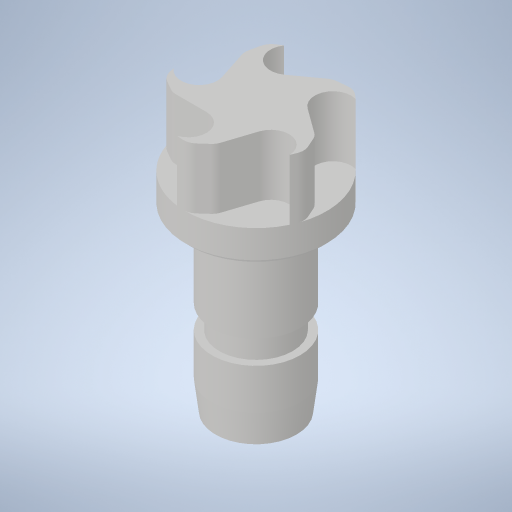
# Autodesk Inventor part: 2.5mm_uncorrected
Saved by Autodesk Inventor 2023.1 (Build 271208000, 208)
## iProperties
Created: 2020-02-22
Part Number: 2.5mm_uncorrected
Material: Generic
Document SubType Name: Modeling
Designer: kongooi
Density: 1 g/cm^3
Appearance: Default
Author: kongooi
Autodesk Inventor part; units mm, degrees
ref_plane "YZ Plane" through (0, 0, 0) normal (1, 0, 0) x (0, 1, 0)
sketch "Sketch2" plane through (0, 0, 0) normal (0, 1, 0) x (-1, 0, 0)
  line L0 (-0.2546, 1.0207) -> (-0.1225, 1.1396)
  line L1 (-0.2546, 1.0207) -> (-0.1225, 1.1396)
  line L2 (-0.3944, -0.9754) -> (-0.571, -0.9938)
  arc A0 (0.5758, -1.0527) -> (0.139, -0.6263) centre (0.3209, -0.8769) ccw
  line L3 (-0.2826, -0.9325) -> (0.139, -0.6263)
  arc A1 (-0.8233, -0.873) -> (-0.7386, -0.9457) centre (-0.0001, 0.0001) ccw
  line L4 (-0.2826, -0.9325) -> (0.139, -0.6263)
  arc A2 (-0.3944, -0.9754) -> (-0.2826, -0.9325) centre (-0.4184, -0.7455) ccw
  line L5 (0.8922, 0.5575) -> (1.046, 0.4685)
  arc A3 (0.1528, 1.1903) -> (0.2557, 0.5886) centre (0.2557, 0.8982) ccw
  line L6 (0.7766, 0.5885) -> (0.2557, 0.5886)
  arc A4 (0.8922, 0.5575) -> (0.7766, 0.5885) centre (0.7766, 0.3574) ccw
  line L7 (0.8057, -0.6769) -> (0.7687, -0.8501)
  arc A5 (1.1791, 0.2224) -> (0.6381, -0.0606) centre (0.9326, 0.035) ccw
  line L8 (0.7994, -0.5574) -> (0.6381, -0.0606)
  arc A6 (0.8057, -0.6769) -> (0.7994, -0.5574) centre (0.5796, -0.6287) ccw
  arc A7 (-1.0848, 0.5133) -> (-0.4808, 0.4252) centre (-0.7752, 0.5209) ccw
  line L9 (-0.3197, 0.9205) -> (-0.4808, 0.4252)
  arc A8 (-0.2546, 1.0207) -> (-0.3197, 0.9205) centre (-0.1, 0.849) ccw
  line L10 (-1.0496, 0.0736) -> (-1.1218, 0.2359)
  arc A9 (-0.8233, -0.873) -> (-0.5529, -0.3258) centre (-0.7349, -0.5763) ccw
  line L11 (-0.9743, -0.0195) -> (-0.5529, -0.3258)
  arc A10 (-1.0496, 0.0736) -> (-0.9743, -0.0195) centre (-0.8385, 0.1675) ccw
  arc A11 (1.1791, 0.2224) -> (1.1534, 0.3311) centre (-0.0001, 0.0001) ccw
  arc A12 (-1.0848, 0.5133) -> (-1.1278, 0.4102) centre (-0.0001, 0.0001) ccw
  arc A13 (0.5758, -1.0527) -> (0.6712, -0.9946) centre (-0.0001, 0.0001) ccw
  arc A14 (0.1528, 1.1903) -> (0.0414, 1.1993) centre (-0.0001, 0.0001) ccw
  arc A15 (0.0414, 1.1993) -> (-0.1225, 1.1396) centre (0.0334, 0.9665) ccw
  arc A16 (-1.1278, 0.4102) -> (-1.1218, 0.2359) centre (-0.9089, 0.3305) ccw
  arc A17 (1.1534, 0.3311) -> (1.046, 0.4685) centre (0.9294, 0.2668) ccw
  arc A18 (-0.7386, -0.9457) -> (-0.571, -0.9938) centre (-0.5953, -0.7621) ccw
  arc A19 (0.6712, -0.9946) -> (0.7687, -0.8501) centre (0.5409, -0.8015) ccw
  circle A20 centre (-0.0001, 0.0001) radius 1.2
  point P0 (-1.0498, 0.074)
  point P1 (0.7767, 0.5884)
  point P2 (0.2555, 0.5884)
  dimension "d305" = 2.4
  constraints: 49 point on circle, 26 tangent, 24 end point, 20 centre point, 12 equal radius, 2 coincident, 2 collinear, 3 other
sketch "Sketch3" plane through (0, 0, 0) normal (0, 1, 0) x (-1, 0, 0)
  line L0 (5.0133, 39.043) -> (38.6813, 7.297)
  line L1 (38.6813, 7.297) -> (18.893, -34.5332)
  line L2 (18.893, -34.5332) -> (-27.0048, -28.6397)
  line L3 (-27.0048, -28.6397) -> (-35.5829, 16.8329)
  line L4 (-35.5829, 16.8329) -> (5.0133, 39.043)
  circle A0 centre (0, 0) radius 39.3635
  circle A1 centre (0, 0) radius 20.4353
  circle A2 centre (0, 0) radius 31.8458
  circle A3 centre (10.4717, -28.7325) radius 10.093
  circle A4 centre (41.1153, -0.5956) radius 4.0726
  circle A5 centre (8.144, 29.3283) radius 10.0252
  circle A6 centre (-25.3778, 16.9956) radius 10.0583
  circle A7 centre (-24.1576, -18.872) radius 10.1582
  line L5 (-25.3778, 16.9956) -> (8.3216, 29.3877)
  line L6 (8.3216, 29.3877) -> (30.5209, 1.1669)
  line L7 (30.5209, 1.1669) -> (10.5413, -28.6665)
  line L8 (10.5413, -28.6665) -> (-24.006, -18.8838)
  line L9 (-24.006, -18.8838) -> (-25.3778, 16.9956)
  line L10 (-31.306, -23.8626) -> (-32.3687, 22.3998)
  line L11 (-32.3687, 22.3998) -> (11.301, 37.7064)
  line L12 (11.301, 37.7064) -> (39.3531, 0.904)
  line L13 (39.3531, 0.904) -> (13.0206, -37.1477)
  line L14 (13.0206, -37.1477) -> (-31.306, -23.8626)
  point P0 (-9.1427, -30.5051)
  constraints: 30 end point, 6 centre point, 6 coincident, 4 tangent, 1 midpoint, 43 other
extrude "Extrusion4" add sketch "Sketch2" against normal blind 1.032 contours L0 A15 A14 A3 L6 A4 L5 A17 A11 A5 L8 A6 L7 A19 A13 A0 L3 A2 L2 A18 A1 A9 L11 A10 L10 A16 A12 A7 L9 A8
sketch "Sketch6" plane through (0, -1.032, 0) normal (0, -1, 0) x (1, 0, 0)
  circle A0 centre (0, 0) radius 1.2
  dimension "d304" = 2.4
  constraints: 1 centre point, 1 coincident
  measures "d304" diameter of A0
extrude "Extrusion5" add sketch "Sketch6" along normal blind 0.55
ref_plane "Plan de construction1" through (0, -1.582, 0) normal (0, -1, 0) x (1, 0, 0)
sketch "Sketch7" plane through (0, -1.582, 0) normal (0, -1, 0) x (1, 0, 0)
  circle A0 centre (0, 0) radius 0.75
  circle A1 centre (0, 0) radius 0.3
  circle A2 centre (0, 0) radius 0.625
  dimension "d303" = 1.5
  dimension "d306" = 0.6
  dimension "d307" = 1.25
  constraints: 3 centre point, 2 coincident
  measures "d303" diameter of A0
  measures "d306" diameter of A1
  measures "d307" diameter of A2
extrude "Extrusion6" add sketch "Sketch7" along normal blind 3 contours A0 | A2
ref_plane "Plan de construction2" through (0, -2.982, 0) normal (0, -1, 0) x (1, 0, 0)
extrude "Extrusion7" cut sketch "Sketch7" along normal blind 0.4 from surface at 1.4 contours A0
chamfer "Chanfrein2" distance 0.5 angle 7 1 edges at (-0.75, -4.582, 0) measured on face at (0.7476, -4.182, -0.0603)
chamfer "Chanfrein3" distance 0.075 angle 45 1 edges at (-1.2, -1.582, 0)
body "Solid4"
